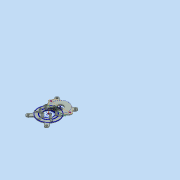
# Autodesk Inventor part: test_rotation
Saved by Autodesk Inventor 2022 (Build 260153000, 153)
## iProperties
Created: 2022-07-27
Part Number: test_rotation
Material: Générique
Document SubType Name: Modeling
Designer: andre
Density: 1 g/cm^3
Appearance: Par défaut(3)
Author: andre
Autodesk Inventor part; units mm, degrees
ref_plane "YZ Plane" through (0, 0, 0) normal (1, 0, 0) x (0, 1, 0)
ref_plane "XZ Plane" through (0, 0, 0) normal (0, 1, 0) x (-1, 0, 0)
sketch "Esquisse1" plane through (0, 0, 0) normal (0, 1, 0) x (-1, 0, 0)
  line L0 (16.5, -7.5) -> (-16.5, -7.5) construction
  line L1 (-16.5, -7.5) -> (-16.5, 7.5) construction
  line L2 (-16.5, 7.5) -> (16.5, 7.5) construction
  line L3 (16.5, 7.5) -> (16.5, -7.5) construction
  circle A0 centre (5, 0) radius 4.7 construction
  circle A1 centre (-5, 0) radius 5.2 construction
  circle A2 centre (0, -26.5) radius 17.5 construction
  line L4 (20.995986, -26.910554) -> (-20.995986, -26.089446) construction
  circle A3 centre (20.995986, -26.910554) radius 2 construction
  circle A4 centre (-20.995986, -26.089446) radius 2 construction
  arc A5 (23.507023, -30.024184) -> (23.626824, -23.897467) centre (20.995986, -26.910554) ccw construction
  arc A6 (-23.507023, -22.975816) -> (-23.626824, -29.102533) centre (-20.995986, -26.089446) ccw construction
  line L5 (-23.626824, -29.102533) -> (-11.509915, -39.682255) construction
  line L6 (-23.507023, -22.975816) -> (-10.985785, -12.877866) construction
  line L7 (23.626824, -23.897467) -> (11.509915, -13.317745) construction
  line L8 (23.507023, -30.024184) -> (10.985785, -40.122134) construction
  circle A7 centre (0, -26.5) radius 4 construction
  line L9 (5, 0) -> (-5, 0) construction
  line L10 (0, 0) -> (0, -26.5) construction
  circle A8 centre (0, 0) radius 10.5 construction
  circle A9 centre (0, 0) radius 22.5
  circle A10 centre (0, 0) radius 15.5
  circle A11 centre (0, 0) radius 15
  circle A12 centre (0, 0) radius 10.5
  circle A13 centre (0, -12.75) radius 2.25
  circle A14 centre (0, -12.75) radius 1
  point P0 (0, 0)
  point P1 (0, -9)
  point P2 (0, -22.5)
  dimension "d19" = 45
  dimension "d0" = 15
  dimension "d1" = 33
  dimension "d2" = 7.5
  dimension "d3" = 7.5
  dimension "d4" = 10
  dimension "d5" = 11.5
  dimension "d6" = 9.4
  dimension "d7" = 10.4
  dimension "d8" = 35
  dimension "d9" = 4
  dimension "d10" = 4
  dimension "d12" = 42
  dimension "d13" = 21
  dimension "d14" = 4
  dimension "d15" = 4
  dimension "d16" = 8
  dimension "d17" = 5
  dimension "d18" = 21
  dimension "d27" = 7
  dimension "d30" = 0.5
  dimension "d31" = 2
  constraints: 22 end point, 14 centre point, 11 coincident, 10 tangent, 9 point on circle, 4 midpoint, 3 point on line, 2 parallel, 1 concentric, 1 horizontal, 1 perpendicular, 1 vertical, 1 vertical alignment, 3 other
  measures "d0" distance of L0.end L1.end
  measures "d1" distance of L1.end L2.end
  measures "d2" distance from line of L2 L9.start
  measures "d3" distance from line of L2 L9.end
  measures "d4" distance of L9.start L9.end
  measures "d5" distance from line of L3 L9.start
  measures "d6" diameter of A0
  measures "d7" diameter of A1
  measures "d8" diameter of A2
  measures "d9" diameter of A3
  measures "d10" diameter of A4
  measures "d12" distance of L4.start L4.end
  measures "d13" distance of L4.start A2.centre
  measures "d14" radius of A5
  measures "d15" radius of A6
  measures "d16" diameter of A7
  measures "d17" distance of L9.end point (0, 0)
  measures "d18" diameter of A8
  measures "d30" radial gap between concentric circles of A10 A11
  measures "d31" diameter of A14
extrude "Extrusion2" add sketch "Esquisse1" along normal blind 8 contours A13
pattern_circular "Réseau circulaire1" count 6 over 360 about axis through (0, 0, 0) along (0, 1, 0) of "Extrusion2"
extrude "Extrusion3" add sketch "Esquisse1" against normal blind 2 contours A9 | A10 | A13 | A11 | A14
ref_plane "Plan de construction2" through (0.043988, 0, -14.99957) normal (-0.0195502, 0, 0.9998089) x (0.9998089, 0, 0.0195502)
ref_plane "Plan de construction1" through (-20.995986, 0, -26.910554) normal (-0.0195502, 0, 0.9998089) x (0.9998089, 0, 0.0195502)
sketch "Esquisse3" plane through (0.043988, 0, -14.99957) normal (-0.0195502, 0, 0.9998089) x (0.9998089, 0, 0.0195502)
  line L0 (0.838755, 1) -> (-0.838755, 1)
  line L1 (9.443432, 0) -> (9.238155, 0)
  arc A0 (1.838755, 0) -> (0.838755, 1) centre (0.838755, 0) ccw
  arc A1 (-0.838755, 1) -> (-1.838755, 0) centre (-0.838755, 0) ccw
  line L2 (2.25, 0) -> (2.25, 8)
  line L3 (-2.25, 0) -> (-2.25, 8)
  line L4 (22.749265, 0) -> (-22.250735, 0)
  point P0 (0.249265, 0)
  point P1 (-0.190614, 0)
  point P2 (0, 1)
  point P3 (1.838755, 0)
  dimension "d40" = 0.83875
  dimension "d41" = 0.83875
  dimension "d42" = 1
  dimension "d43" = 2.25
  dimension "d44" = 2.25
  constraints: 4 point on circle, 2 centre point, 2 end point, 2 tangent, 1 horizontal, 1 line through centre, 1 midpoint, 1 point on line, 3 other
  measures "d40" distance of L0.end point (0, 1)
  measures "d41" distance of L0.start point (0, 1)
  measures "d42" distance of the line from the sketch origin of L0
  measures "d43" distance from line of L2 point (0, 1)
  measures "d44" distance from line of L3 point (0, 1)
extrude "Extrusion4" add sketch "Esquisse3" along normal up to surface round surface about axis through (0, 0, -12.75) along (0, 1, 0) radius 2.25 far side no
extrude "Extrusion5" add sketch "Esquisse3" against normal up to surface round surface about axis through (0, 0, 0) along (0, -1, 0) radius 22.5 far side no
pattern_circular "Réseau circulaire2" count 6 over 360 about axis through (0, 0, 0) along (0, 1, 0) of "Extrusion4", "Extrusion5"
sketch "Esquisse4" plane through (0, 0, 0) normal (0, 1, 0) x (1, 0, 0)
  line L0 (23.626824, 29.102533) -> (11.509915, 39.682255) construction
  circle A0 centre (0, 26.5) radius 17.5 construction
  line L1 (-23.507023, 30.024184) -> (-10.985785, 40.122134) construction
  arc A1 (-23.507023, 30.024184) -> (-23.626824, 23.897467) centre (-20.995986, 26.910554) ccw construction
  arc A2 (23.507023, 22.975816) -> (23.626824, 29.102533) centre (20.995986, 26.089446) ccw construction
  line L2 (23.507023, 22.975816) -> (10.985785, 12.877866) construction
  line L3 (-23.626824, 23.897467) -> (-11.509915, 13.317745) construction
  circle A3 centre (0, 0) radius 22.5
  arc A4 (23.507023, 22.975816) -> (20.388259, 9.51677) centre (30.539829, 14.255289) ccw
  arc A5 (23.507023, 22.975816) -> (23.626824, 29.102533) centre (20.995986, 26.089446) ccw
  line L4 (23.626824, 29.102533) -> (11.509915, 39.682255)
  arc A6 (11.509915, 39.682255) -> (-10.985785, 40.122134) centre (0, 26.5) ccw
  line L5 (-10.985785, 40.122134) -> (-23.507023, 30.024184)
  arc A7 (-23.507023, 30.024184) -> (-23.626824, 23.897467) centre (-20.995986, 26.910554) ccw
  arc A8 (-20.477012, 9.324268) -> (-23.626824, 23.897467) centre (-31.835324, 14.496308) ccw
  circle A9 centre (20.995986, 26.089446) radius 2
  circle A10 centre (-20.995986, 26.910554) radius 2
  constraints: 12 point on circle, 7 tangent, 5 centre point, 4 end point, 3 coincident, 1 collinear
extrude "Extrusion6" add sketch "Esquisse4" against normal up to surface (2 mm away) contours A3 A8 A7 L5 A6 L4 A5 A4
sketch "Esquisse5" plane through (0, 0, 0) normal (0, 1, 0) x (1, 0, 0)
  circle A0 centre (0, 26.5) radius 6
  point P0 (0, 0)
  dimension "d54" = 12
  constraints: 1 centre point, 1 coincident
  measures "d54" diameter of A0
extrude "Extrusion7" cut sketch "Esquisse5" along normal through all both and the other way through all
sketch "Esquisse6" plane through (0, 0, 0) normal (0, 1, 0) x (1, 0, 0)
  circle A0 centre (20, 38.906959) radius 2
  arc A1 (23.013087, 36.276121) -> (16.986913, 41.537796) centre (20, 38.906959) ccw
  line L0 (23.013087, 36.276121) -> (19.72454, 32.509762)
  line L1 (11.509915, 39.682255) -> (23.626824, 29.102533)
  line L2 (16.986913, 41.537796) -> (13.538646, 37.588511)
  arc A2 (11.509915, 39.682255) -> (-10.985785, 40.122134) centre (0, 26.5) ccw
  line L3 (0, -75.321489) -> (0, -45.506687)
  circle A3 centre (-20, 38.906959) radius 2
  arc A4 (-16.986913, 41.537796) -> (-23.013087, 36.276121) centre (-20, 38.906959) ccw
  line L4 (-23.013087, 36.276121) -> (-19.72454, 32.509762)
  line L5 (-16.986913, 41.537796) -> (-13.538646, 37.588511)
  line L6 (20, 38.906959) -> (20, -65.992975)
  line L7 (-20, 38.906959) -> (-20, -70.59957)
  circle A5 centre (20, -23.685439) radius 2
  arc A6 (16.943814, -26.266084) -> (23.056186, -21.104793) centre (20, -23.685439) ccw
  line L8 (23.056186, -21.104793) -> (17.341082, -14.336557)
  line L9 (16.943814, -26.266084) -> (11.228711, -19.497847)
  arc A7 (-20.477012, 9.324268) -> (20.388259, 9.51677) centre (0, 0) ccw
  line L10 (20, -23.685439) -> (0, 0)
  arc A8 (1.64964, -22.439445) -> (18.392279, -12.960481) centre (0, 0) ccw
  circle A9 centre (-20, -23.685439) radius 2
  arc A10 (-23.056186, -21.104793) -> (-16.943814, -26.266084) centre (-20, -23.685439) ccw
  line L11 (-23.056186, -21.104793) -> (-17.341082, -14.336557)
  line L12 (-16.943814, -26.266084) -> (-11.228711, -19.497847)
  line L13 (-23.507023, 30.024184) -> (-10.985785, 40.122134) construction
  line L14 (-23.507023, 30.024184) -> (-10.985785, 40.122134)
  line L15 (-13.781928, 37.867141) -> (-20, 32.852478)
  point P0 (13.698366, 37.771438)
  point P1 (-20.013953, 32.841226)
  dimension "d57" = 4
  dimension "d58" = 8
  dimension "d59" = 5
  dimension "d60" = 40
  dimension "d61" = 8
  dimension "d62" = 4
  dimension "d63" = 31
  constraints: 26 end point, 12 symmetric about line, 11 point on circle, 8 centre point, 7 point on line, 4 coincident, 4 tangent, 3 vertical, 2 parallel, 2 perpendicular, 4 other
  measures "d57" diameter of A0
  measures "d58" diameter of A1
  measures "d59" distance from line of L1 L6.start
  measures "d60" distance of A4.centre A0.centre
  measures "d61" diameter of A6
  measures "d62" diameter of A5
  measures "d63" distance of A7.centre A5.centre
extrude "Extrusion8" add sketch "Esquisse6" against normal up to surface (2 mm away) contours L0 L1 L2 A1 | L8 A6 L6 A5 | L6 A5 L10 A7 L8 | L14 L4 A4 L5 | A5 L6 A6 L9 A7 L10 | L11 A7 L12 A10 L7 A9 | L7 A9 A10 L11
fillet "Congé1" radius 3 8 edges at (13.6984, -1, -37.7714) (19.7245, -1, -32.5098) (17.3411, -1, 14.3366) (11.2287, -1, 19.4978) (-11.2287, -1, 19.4978) (-17.3411, -1, 14.3366) (-20.014, -1, -32.8412) (-13.7819, -1, -37.8671)
equation "\"d5\" = -0.5 * d4 + 0.5 * d1"
equation "\"d13\" = 0.5 * d12"
equation "\"d17\" = 0.5 * d4"
